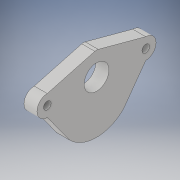
# Autodesk Inventor part: MotorFixedPositionMount
Saved by Autodesk Inventor 2017 (Build 210142000, 142)
## iProperties
Created: 2017-08-12
Part Number: MotorFixedPositionMount
Material: Generic
Document SubType Name: Modeling
Designer: User
Density: 1 g/cm^3
Appearance: Default
Author: User
Autodesk Inventor part; units mm, degrees
ref_plane "YZ Plane" through (0, 0, 0) normal (1, 0, 0) x (0, 1, 0)
ref_plane "XZ Plane" through (0, 0, 0) normal (0, 1, 0) x (-1, 0, 0)
ref_plane "XY Plane" through (0, 0, 0) normal (0, 0, 1) x (1, 0, 0)
sketch "Sketch1" plane through (0, 0, 0) normal (1, 0, 0) x (0, 1, 0)
  circle A0 centre (7.0104, 24.0085) radius 1.8542
  circle A1 centre (7.0104, -23.9975) radius 1.8542
  arc A2 (12.0396, 24.0085) -> (1.9812, 24.0085) centre (7.0104, 24.0085) ccw
  arc A3 (1.9812, -23.9975) -> (12.0396, -23.9975) centre (7.0104, -23.9975) ccw
  line L0 (12.0396, 24.0085) -> (18.5, 0.0055)
  line L1 (12.0396, -23.9975) -> (18.5, 0.0055)
  line L2 (1.9812, 24.0085) -> (-13.0815, 13.087)
  line L3 (-13.0815, -13.0759) -> (1.9812, -23.9975)
  arc A4 (-13.0815, 13.087) -> (-13.0815, -13.0759) centre (0, 0.0055) ccw
  circle A5 centre (7, 0) radius 6.0325
  point P0 (0, 0)
  dimension "d8" = 3.7084
  dimension "d11" = 3.7084
  dimension "d14" = 10.0584
  dimension "d15" = 10.0584
  constraints: 8 end point, 6 centre point, 6 point on circle, 2 coincident
  measures "d8" diameter of A0
  measures "d11" diameter of A1
  measures "d14" diameter of A2
  measures "d15" diameter of A3
extrude "Extrusion1" add sketch "Sketch1" along normal blind 6.35
fillet "Fillet1" radius 3.175 1 edges at (3.175, 18.5, 0.0055)
body "Solid1"
